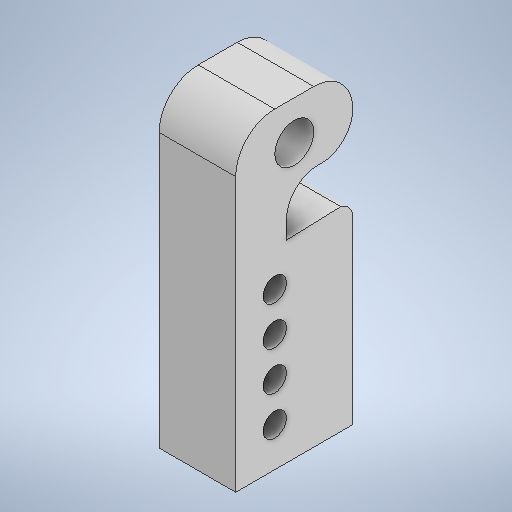
# Autodesk Inventor part: ReleasePin
Saved by Autodesk Inventor 2025 (Build 290162000, 162)
## iProperties
Created: 2025-11-05
Part Number: ReleasePin
Material: Generic
Document SubType Name: Modeling
Designer: ruven
Density: 1 g/cm^3
Appearance: Default
Author: ruven
Autodesk Inventor part; units mm, degrees
ref_plane "YZ Plane" through (0, 0, 0) normal (1, 0, 0) x (0, 1, 0)
ref_plane "XZ Plane" through (0, 0, 0) normal (0, 1, 0) x (-1, 0, 0)
ref_plane "XY Plane" through (0, 0, 0) normal (0, 0, 1) x (1, 0, 0)
sketch "Sketch1" plane through (0, 0, 0) normal (1, 0, 0) x (0, 1, 0)
  line L0 (-20, -7.5) -> (20, -7.5)
  line L1 (20, -7.5) -> (20, 7.5)
  line L2 (20, 7.5) -> (-20, 7.5)
  line L3 (-20, 7.5) -> (-20, -7.5)
  line L4 (-20, -7.5) -> (20, 7.5) construction
  line L5 (20, -7.5) -> (-20, 7.5) construction
  point P0 (0, 0)
  dimension "d0" = 15
  dimension "d1" = 40
  constraints: 12 end point, 2 midpoint, 2 parallel, 1 horizontal, 1 perpendicular
  measures "d0" distance of L0.end L1.end
  measures "d1" distance of L1.end L2.end
extrude "Extrusion1" add sketch "Sketch1" along normal blind 5
sketch "Sketch2" plane through (5, 0, 0) normal (1, 0, 0) x (0, 0, -1)
  circle A0 centre (0, 15) radius 2.5
  line L0 (7.5, 20) -> (-7.5, 20) projected
  line L1 (7.5, -20) -> (7.5, 20) projected
  point P0 (0, 0)
  dimension "d4" = 5
  dimension "d5" = 5
  dimension "d7" = 7.5
  constraints: 1 centre point
  measures "d4" diameter of A0
  measures "d5" distance from line of L0 A0.centre
  measures "d7" distance from line of L1 A0.centre
fillet "Fillet1" radius 5 2 edges at (2.5, 20, -7.5) (2.5, 20, 7.5)
extrude "Extrusion2" cut sketch "Sketch2" against normal blind 5
sketch "Sketch3" plane through (5, 0, 0) normal (1, 0, 0) x (0, 0, -1)
  line L0 (7.5, -20) -> (7.5, 15) projected
  line L1 (7.5, 11) -> (-1, 11)
  line L2 (-1, 11) -> (-1, 5)
  line L3 (-1, 5) -> (7.5, 5)
  line L4 (7.5, 5) -> (7.5, 11)
  circle A0 centre (0, 15) radius 2.5 projected
  point P0 (0, 0)
  point P1 (7.5, 5)
  dimension "d10" = 4
  dimension "d12" = 1
  dimension "d18" = 10
  constraints: 8 end point, 2 parallel, 1 horizontal, 1 perpendicular, 1 point on line
  measures "d10" distance from line of L1 A0.centre
  measures "d12" distance from line of A0.centre L2
  measures "d18" distance from line of L3 A0.centre
extrude "Extrusion3" cut sketch "Sketch3" against normal blind 10 contours L3 L2 L1 L0
fillet "Fillet2" radius 4 2 edges at (2.5, 11, 1) (2.5, 11, -7.5)
fillet "Fillet3" radius 2 1 edges at (2.5, 5, -7.5)
sketch "Sketch4" plane through (5, 0, 0) normal (1, 0, 0) x (0, 0, -1)
  line L0 (-1, 5) -> (5.5, 5) projected
  line L1 (-1, 5) -> (7.5, 5)
  line L2 (7.5, 5) -> (-1, 4.7032)
  line L3 (-1, 4.7032) -> (-1, 5)
  point P0 (0, 0)
  dimension "d20" = 2
  constraints: 6 end point, 1 horizontal, 1 perpendicular
  measures "d20" angle of L2 L0
extrude "Extrusion4" cut sketch "Sketch4" against normal blind 10
sketch "Sketch5" plane through (5, 0, 0) normal (1, 0, 0) x (0, 0, -1)
  line L0 (-1, 4.7032) -> (-1, 7) projected
  arc A0 (3, 11) -> (-1, 7) centre (3, 7) ccw projected
  line L1 (3, 11) -> (3.5, 11) projected
  arc A1 (3.5, 11) -> (7.5, 15) centre (3.5, 15) ccw projected
  arc A2 (7.5, 15) -> (2.5, 20) centre (2.5, 15) ccw projected
  line L2 (2.5, 20) -> (-2.5, 20) projected
  arc A3 (-2.5, 20) -> (-7.5, 15) centre (-2.5, 15) ccw projected
  line L3 (-7.5, 15) -> (-7.5, -20) projected
  line L4 (-7.5, -20) -> (7.5, -20) projected
  line L5 (7.5, -20) -> (7.5, 3) projected
  arc A4 (7.5, 3) -> (5.9606, 4.9462) centre (5.5, 3) ccw projected
  line L6 (5.9606, 4.9462) -> (-1, 4.7032) projected
  circle A5 centre (0, 15) radius 2.5 projected
  point P0 (0, 0)
extrude "Extrusion5" add sketch "Sketch5" along normal blind 1.5
sketch "Sketch6" plane through (6.5, 0, 0) normal (1, 0, 0) x (0, 0, -1)
  circle A0 centre (-2.5, -15) radius 1.5
  line L0 (-7.5, -20) -> (7.5, -20) projected
  line L1 (-7.5, 15) -> (-7.5, -20) projected
  circle A1 centre (-2.5, 0) radius 1.5
  circle A2 centre (-2.5, -5) radius 1.5
  circle A3 centre (-2.5, -10) radius 1.5
  point P0 (0, 0)
  dimension "d25" = 3
  dimension "d26" = 5
  dimension "d27" = 5
  dimension "d32" = 3
  dimension "d33" = 20
  dimension "d34" = 3
  dimension "d35" = 3
  dimension "d36" = 10
  dimension "d37" = 15
  constraints: 4 centre point
  measures "d25" diameter of A0
  measures "d26" distance from line of L0 A0.centre
  measures "d27" distance from line of L1 A0.centre
  measures "d32" diameter of A1
  measures "d33" distance from line of L0 A1.centre
  measures "d34" diameter of A2
  measures "d35" diameter of A3
  measures "d36" distance from line of A3.centre L0
  measures "d37" distance from line of L0 A2.centre
extrude "Extrusion6" cut sketch "Sketch6" against normal through all
sketch "Sketch7" plane through (0, 0, 0) normal (-1, 0, 0) x (0, 0, 1)
  circle A0 centre (2.5, -15) radius 1.5 projected
  circle A1 centre (0, 15) radius 2.5 projected
  line L0 (1, 7) -> (1, 4.7032) projected
  line L1 (1, 4.7032) -> (-5.9606, 4.9462) projected
  arc A2 (-5.9606, 4.9462) -> (-7.5, 3) centre (-5.5, 3) ccw projected
  line L2 (-7.5, -20) -> (-7.5, 3) projected
  line L3 (7.5, -20) -> (-7.5, -20) projected
  line L4 (7.5, 15) -> (7.5, -20) projected
  arc A3 (7.5, 15) -> (2.5, 20) centre (2.5, 15) ccw projected
  line L5 (-2.5, 20) -> (2.5, 20) projected
  arc A4 (-2.5, 20) -> (-7.5, 15) centre (-2.5, 15) ccw projected
  arc A5 (-7.5, 15) -> (-3.5, 11) centre (-3.5, 15) ccw projected
  line L6 (-3.5, 11) -> (-3, 11) projected
  arc A6 (1, 7) -> (-3, 11) centre (-3, 7) ccw projected
  point P0 (0, 0)
extrude "Extrusion7" add sketch "Sketch7" along normal blind 3.3
body "Solid1"
